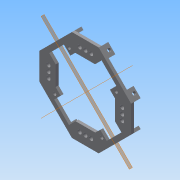
# Autodesk Inventor part: fix_board
Saved by Autodesk Inventor 2015 (Build 190159000, 159)
## iProperties
Created: 2015-06-18
Part Number: fix_board
Material: Générique
Document SubType Name: Modeling
Designer: Gregwar
Density: 1 g/cm^3
Appearance: Par défaut
Author: Gregwar
Autodesk Inventor part; units mm, degrees
note: some values were not read from the file. Chosen so that the rebuilt part matches the saved one: second side of "Extrusion3".
ref_plane "YZ Plane" through (0, 0, 0) normal (1, 0, 0) x (0, 1, 0)
ref_plane "XZ Plane" through (0, 0, 0) normal (0, 1, 0) x (-1, 0, 0)
ref_plane "XY Plane" through (0, 0, 0) normal (0, 0, 1) x (1, 0, 0)
sketch "Esquisse1" plane through (0, 0, 0) normal (0, 1, 0) x (-1, 0, 0)
  line L0 (35, 35) -> (35, 14)
  line L1 (35, 14) -> (42, 10)
  line L2 (42, 10) -> (42, 0)
  line L3 (35, 35) -> (0, 0)
  line L4 (42, 0) -> (0, 0) construction
  line L5 (35, -35) -> (35, -14)
  line L6 (35, -14) -> (42, -10)
  line L7 (42, -10) -> (42, 0)
  line L8 (35, -35) -> (0, 0)
  line L9 (38.5, -12) -> (38.5, 12) construction
  circle A0 centre (38.5, 0) radius 2.15
  circle A1 centre (38.5, 6) radius 2.15
  circle A2 centre (38.5, -6) radius 2.15
  dimension "d0" = 90
  dimension "d1" = 70
  dimension "d4" = 6
  dimension "d11" = 6
  dimension "d16" = 4.3
  dimension "d17" = 20
  dimension "d18" = 4
  dimension "d19" = 7
  constraints: 20 end point, 3 centre point, 3 midpoint, 3 symmetric about line, 3 vertical, 1 horizontal, 1 parallel, 4 other
  measures "d0" angle of L3 L8
  measures "d1" distance of L0.start L5.start
  measures "d4" distance of A0.centre A1.centre
  measures "d11" distance of A0.centre A2.centre
  measures "d16" diameter of A0
  measures "d17" distance of L1.end L6.end
  measures "d18" vertical distance of L1.end L0.end
  measures "d19" distance between parallel lines of L5 L7
extrude "Extrusion1" add sketch "Esquisse1" along normal blind 3
pattern_circular "Réseau circulaire1" count 4 over 360 about axis through (0, 0, 0) along (0, 1, 0) of "Extrusion1"
chamfer "Chanfrein1" distance 8 angle 45 4 edges at (35, 1.5, -35) (-35, 1.5, -35) (-35, 1.5, 35) (35, 1.5, 35)
ref_plane "Plan de construction3" through (-4, 0, 4) normal (0.7071068, 0, 0.7071068) x (0.7071068, 0, -0.7071068)
ref_plane "Plan de construction4" through (-4, 0, -4) normal (-0.7071068, 0, 0.7071068) x (0.7071068, 0, 0.7071068)
sketch "Esquisse3" plane through (0, 0, 0) normal (0, -1, 0) x (1, 0, 0)
  circle A0 centre (0, 38.5) radius 2.15 projected
  circle A1 centre (6, 38.5) radius 2.15 projected
  circle A2 centre (-6, 38.5) radius 2.15 projected
  circle A3 centre (38.5, 6) radius 2.15 projected
  circle A4 centre (38.5, -6) radius 2.15 projected
  circle A5 centre (38.5, 0) radius 2.15 projected
  circle A6 centre (6, -38.5) radius 2.15 projected
  circle A7 centre (-6, -38.5) radius 2.15 projected
  circle A8 centre (0, -38.5) radius 2.15 projected
  circle A9 centre (-38.5, -6) radius 2.15 projected
  circle A10 centre (-38.5, 6) radius 2.15 projected
  circle A11 centre (-38.5, 0) radius 2.15 projected
  line L0 (27, 35) -> (35, 27) projected
  line L1 (27, 35) -> (14, 35) projected
  line L2 (14, 35) -> (10, 42) projected
  line L3 (10, 42) -> (-10, 42) projected
  line L4 (-10, 42) -> (-14, 35) projected
  line L5 (-14, 35) -> (-27, 35) projected
  line L6 (-35, 27) -> (-27, 35) projected
  line L7 (-35, 27) -> (-35, 14) projected
  line L8 (-35, 14) -> (-42, 10) projected
  line L9 (-42, 10) -> (-42, -10) projected
  line L10 (-42, -10) -> (-35, -14) projected
  line L11 (-35, -14) -> (-35, -27) projected
  line L12 (-27, -35) -> (-35, -27) projected
  line L13 (-27, -35) -> (-14, -35) projected
  line L14 (-14, -35) -> (-10, -42) projected
  line L15 (-10, -42) -> (10, -42) projected
  line L16 (10, -42) -> (14, -35) projected
  line L17 (14, -35) -> (27, -35) projected
  line L18 (35, -27) -> (27, -35) projected
  line L19 (35, -27) -> (35, -14) projected
  line L20 (35, -14) -> (42, -10) projected
  line L21 (42, -10) -> (42, 10) projected
  line L22 (42, 10) -> (35, 14) projected
  line L23 (35, 14) -> (35, 27) projected
  line L24 (-47.9706, 14.0294) -> (-14.0294, 47.9706)
  line L25 (-14.0294, 47.9706) -> (-11.9081, 45.8492)
  line L26 (-11.9081, 45.8492) -> (-45.8492, 11.9081)
  line L27 (-45.8492, 11.9081) -> (-47.9706, 14.0294)
  point P0 (0, 0)
  point P1 (-31, 31)
  dimension "d35" = 48
  dimension "d36" = 3
  constraints: 8 end point, 2 midpoint, 2 perpendicular, 1 collinear, 1 parallel
  measures "d35" distance of L24.start L24.end
  measures "d36" distance of L24.end L25.end
extrude "Extrusion3" add sketch "Esquisse3" against normal blind 10 contours L26 L7 L6 L5 | L5 L24 L25 L26 | L26 L27 L24 L7
sketch "Esquisse4" plane through (-14.0294, 0, 47.9706) normal (-0.7071068, 0, 0.7071068) x (0.7071068, 0, 0.7071068)
  line L0 (0, 0) -> (-48, 0) projected
  line L1 (0, 0) -> (0, 10) projected
  line L2 (-48, 10) -> (0, 10) projected
  line L3 (-48, 0) -> (-48, 10) projected
  line L4 (-48, 0) -> (-48, 10) construction
  line L5 (-48, 7) -> (0, 7) construction
  line L6 (0, 0) -> (0, 10) construction
  circle A0 centre (-42.5, 7) radius 1.75
  line L7 (0, 10) -> (-48, 10) construction
  line L8 (-24, 10) -> (-24, 0) construction
  circle A1 centre (-5.5, 7) radius 1.75
  dimension "d41" = 10
  dimension "d42" = 3
  dimension "d43" = 37
  dimension "d44" = 3.5
  constraints: 4 end point, 3 point on line, 2 centre point, 1 horizontal, 1 midpoint, 1 symmetric about line, 1 vertical, 1 other
  measures "d41" distance between parallel lines of L0 L2
  measures "d42" distance between parallel lines of L5 L2
  measures "d43" distance of A0.centre A1.centre
  measures "d44" diameter of A0
extrude "Extrusion4" cut sketch "Esquisse4" against normal through all contours A0 | A1
sketch "Esquisse6" plane through (-14.0294, 0, 47.9706) normal (-0.7071068, 0, 0.7071068) x (0.7071068, 0, 0.7071068)
  line L0 (-15.3431, 3) -> (-9.1508, 3) projected
  circle A0 centre (-5.5, 7) radius 1.75 projected
  circle A1 centre (-42.5, 7) radius 1.75 projected
  line L1 (0, 0) -> (-48, 0) projected
  line L2 (0, 0) -> (0, 10) projected
  line L3 (-48, 10) -> (0, 10) projected
  line L4 (-48, 0) -> (-48, 10) projected
  line L5 (-10.5, 10) -> (-37.5, 10)
  line L6 (-37.5, 10) -> (-37.5, 3)
  line L7 (-37.5, 3) -> (-10.5, 3)
  line L8 (-10.5, 3) -> (-10.5, 10)
  point P0 (-24, 0)
  point P1 (-24, 10)
  dimension "d51" = 27
  dimension "d63" = 3
  constraints: 8 end point, 2 midpoint, 2 parallel, 1 horizontal, 1 perpendicular
  measures "d51" distance of L6.end L7.end
  measures "d63" distance between parallel lines of L7 L1
extrude "Extrusion5" cut sketch "Esquisse6" against normal through all contours L7 L6 L3 L8 L0
pattern_circular "Réseau circulaire5" count 4 over 360 about axis through (0, 0, 0) along (0, 1, 0) of "Extrusion3", "Extrusion4", "Extrusion5"
sketch "Esquisse11" plane through (0, 0, 0) normal (0, -1, 0) x (1, 0, 0)
  circle A0 centre (0, 38.5) radius 2.15 construction
  circle A1 centre (6, 38.5) radius 2.15 construction
  circle A2 centre (-6, 38.5) radius 2.15 construction
  circle A3 centre (38.5, 6) radius 2.15 construction
  circle A4 centre (38.5, -6) radius 2.15 construction
  circle A5 centre (38.5, 0) radius 2.15 construction
  circle A6 centre (6, -38.5) radius 2.15 construction
  circle A7 centre (-6, -38.5) radius 2.15 construction
  circle A8 centre (0, -38.5) radius 2.15 construction
  circle A9 centre (-38.5, -6) radius 2.15 construction
  circle A10 centre (-38.5, 6) radius 2.15 construction
  circle A11 centre (-38.5, 0) radius 2.15 construction
  line L0 (-22.7574, -35) -> (-14, -35) construction
  line L1 (-14, -35) -> (-10, -42) construction
  line L2 (-10, -42) -> (10, -42) construction
  line L3 (10, -42) -> (14, -35) construction
  line L4 (14, -35) -> (22.7574, -35) construction
  line L5 (22.7574, -35) -> (11.9081, -45.8492) construction
  line L6 (11.9081, -45.8492) -> (14.0294, -47.9706) construction
  line L7 (14.0294, -47.9706) -> (47.9706, -14.0294) construction
  line L8 (47.9706, -14.0294) -> (45.8492, -11.9081) projected
  line L9 (45.8492, -11.9081) -> (35, -22.7574) projected
  line L10 (35, -22.7574) -> (35, -14) projected
  line L11 (35, -14) -> (42, -10) projected
  line L12 (42, -10) -> (42, 10) projected
  line L13 (42, 10) -> (35, 14) projected
  line L14 (35, 14) -> (35, 22.7574) projected
  line L15 (35, 22.7574) -> (45.8492, 11.9081) projected
  line L16 (45.8492, 11.9081) -> (47.9706, 14.0294) projected
  line L17 (47.9706, 14.0294) -> (14.0294, 47.9706) construction
  line L18 (14.0294, 47.9706) -> (11.9081, 45.8492) construction
  line L19 (11.9081, 45.8492) -> (22.7574, 35) construction
  line L20 (22.7574, 35) -> (14, 35) construction
  line L21 (14, 35) -> (10, 42) construction
  line L22 (10, 42) -> (-10, 42) construction
  line L23 (-10, 42) -> (-14, 35) construction
  line L24 (-14, 35) -> (-22.7574, 35) construction
  line L25 (-22.7574, 35) -> (-11.9081, 45.8492) construction
  line L26 (-11.9081, 45.8492) -> (-14.0294, 47.9706) construction
  line L27 (-14.0294, 47.9706) -> (-47.9706, 14.0294) construction
  line L28 (-47.9706, 14.0294) -> (-45.8492, 11.9081) construction
  line L29 (-45.8492, 11.9081) -> (-35, 22.7574) construction
  line L30 (-35, 22.7574) -> (-35, 14) construction
  line L31 (-35, 14) -> (-42, 10) construction
  line L32 (-42, 10) -> (-42, -10) construction
  line L33 (-42, -10) -> (-35, -14) construction
  line L34 (-35, -14) -> (-35, -22.7574) construction
  line L35 (-35, -22.7574) -> (-45.8492, -11.9081) construction
  line L36 (-45.8492, -11.9081) -> (-47.9706, -14.0294) construction
  line L37 (-47.9706, -14.0294) -> (-14.0294, -47.9706) construction
  line L38 (-14.0294, -47.9706) -> (-11.9081, -45.8492) construction
  line L39 (-11.9081, -45.8492) -> (-22.7574, -35) construction
  line L40 (47.9706, -14.0294) -> (47.9706, 14.0294)
  point P0 (0, 0)
  constraints: 2 end point, 1 vertical
extrude "Extrusion8" add sketch "Esquisse11" against normal blind 3
pattern_circular "Réseau circulaire6" count 4 over 360 about axis through (0, 0, 0) along (0, 1, 0) of "Extrusion8"
sketch "Esquisse9" plane through (0, 0, 0) normal (0, -1, 0) x (1, 0, 0)
  line L0 (0, 0) -> (21.8388, 21.8388) construction
  line L1 (0, 0) -> (66.7346, 0) construction
  line L2 (0, 0) -> (0, 22.6965) construction
  line L3 (31.4289, 0) -> (31.4289, 10)
  line L4 (31.4289, 10) -> (38.5, 17.0711)
  line L5 (38.5, 17.0711) -> (27.7855, 27.7855)
  line L6 (0, 31.4289) -> (10, 31.4289)
  line L7 (10, 31.4289) -> (17.0711, 38.5)
  line L8 (17.0711, 38.5) -> (27.7855, 27.7855)
  line L9 (38.5, -17.0711) -> (27.7855, -27.7855)
  line L10 (31.4289, -10) -> (38.5, -17.0711)
  line L11 (31.4289, 0) -> (31.4289, -10)
  line L12 (17.0711, -38.5) -> (27.7855, -27.7855)
  line L13 (10, -31.4289) -> (17.0711, -38.5)
  line L14 (0, -31.4289) -> (10, -31.4289)
  line L15 (-31.4289, 0) -> (-31.4289, -10)
  line L16 (-31.4289, -10) -> (-38.5, -17.0711)
  line L17 (-38.5, -17.0711) -> (-27.7855, -27.7855)
  line L18 (-17.0711, -38.5) -> (-27.7855, -27.7855)
  line L19 (0, -31.4289) -> (-10, -31.4289)
  line L20 (-10, -31.4289) -> (-17.0711, -38.5)
  line L21 (0, 0) -> (-66.7346, 0) construction
  line L22 (-31.4289, 0) -> (-31.4289, 10)
  line L23 (-31.4289, 10) -> (-38.5, 17.0711)
  line L24 (0, 31.4289) -> (-10, 31.4289)
  line L25 (0, 0) -> (-21.8388, 21.8388) construction
  line L26 (-10, 31.4289) -> (-17.0711, 38.5)
  line L27 (-17.0711, 38.5) -> (-27.7855, 27.7855)
  line L28 (-38.5, 17.0711) -> (-27.7855, 27.7855)
  line L29 (27.432, 27.432) -> (37.7929, 17.0711)
  line L30 (37.7929, 17.0711) -> (30.9289, 10.2071)
  line L31 (30.9289, 10.2071) -> (30.9289, 0)
  line L32 (30.9289, 0) -> (30.9289, -10.2071)
  line L33 (30.9289, -10.2071) -> (37.7929, -17.0711)
  line L34 (37.7929, -17.0711) -> (27.432, -27.432)
  line L35 (27.432, -27.432) -> (17.0711, -37.7929)
  line L36 (17.0711, -37.7929) -> (10.2071, -30.9289)
  line L37 (10.2071, -30.9289) -> (0, -30.9289)
  line L38 (0, -30.9289) -> (-10.2071, -30.9289)
  line L39 (-10.2071, -30.9289) -> (-17.0711, -37.7929)
  line L40 (-17.0711, -37.7929) -> (-27.432, -27.432)
  line L41 (-27.432, -27.432) -> (-37.7929, -17.0711)
  line L42 (-37.7929, -17.0711) -> (-30.9289, -10.2071)
  line L43 (-30.9289, -10.2071) -> (-30.9289, 0)
  line L44 (-30.9289, 0) -> (-30.9289, 10.2071)
  line L45 (-30.9289, 10.2071) -> (-37.7929, 17.0711)
  line L46 (-37.7929, 17.0711) -> (-27.432, 27.432)
  line L47 (-27.432, 27.432) -> (-17.0711, 37.7929)
  line L48 (-17.0711, 37.7929) -> (-10.2071, 30.9289)
  line L49 (-10.2071, 30.9289) -> (0, 30.9289)
  line L50 (0, 30.9289) -> (10.2071, 30.9289)
  line L51 (10.2071, 30.9289) -> (17.0711, 37.7929)
  line L52 (17.0711, 37.7929) -> (27.432, 27.432)
  dimension "d67" = 45
  dimension "d68" = 10
  dimension "d69" = 10
  dimension "d70" = 38.5
  dimension "d71" = 77
  dimension "d86" = 0.5
  constraints: 106 end point, 22 symmetric about line, 4 point on line, 2 collinear, 2 parallel, 2 vertical, 1 coincident, 1 horizontal, 23 other
  measures "d67" angle of L0 L1
  measures "d68" distance of L3.start L3.end
  measures "d69" distance of L3.end L5.start
  measures "d70" distance from line of L1 L7.end
  measures "d71" distance of L13.end L7.end
  measures "d86" distance between parallel lines of L5 L29
extrude "Extrusion9" cut sketch "Esquisse9" against normal through all contours L29 L30 L31 L32 L33 L34 L35 L36 L37 L38 L39 L40 L41 L42 L43 L44 L45 L46 L47 L48 L49 L50 L51 L52
sketch "Esquisse12" plane through (0, 3, 0) normal (0, 1, 0) x (1, 0, 0)
  line L0 (-10, -31.4289) -> (-17.0711, -38.5) projected
  line L1 (-17.0711, -38.5) -> (-27.7855, -27.7855) projected
  line L2 (-31.4289, -10) -> (-38.5, -17.0711) projected
  line L3 (-38.5, -17.0711) -> (-27.7855, -27.7855) projected
  line L4 (-10, -31.4289) -> (-15.6569, -25.7721)
  line L5 (-15.6569, -25.7721) -> (-22.7279, -32.8431)
  circle A0 centre (-17.0711, -32.136) radius 1.75
  line L6 (-10, -31.4289) -> (-17.0711, -38.5)
  line L7 (-17.0711, -38.5) -> (-22.7279, -32.8431)
  line L8 (31.4289, -10) -> (25.7721, -15.6569)
  line L9 (25.7721, -15.6569) -> (32.8431, -22.7279)
  circle A1 centre (32.136, -17.0711) radius 1.75
  line L10 (31.4289, -10) -> (38.5, -17.0711)
  line L11 (38.5, -17.0711) -> (32.8431, -22.7279)
  line L12 (10, 31.4289) -> (15.6569, 25.7721)
  line L13 (15.6569, 25.7721) -> (22.7279, 32.8431)
  circle A2 centre (17.0711, 32.136) radius 1.75
  line L14 (10, 31.4289) -> (17.0711, 38.5)
  line L15 (17.0711, 38.5) -> (22.7279, 32.8431)
  line L16 (-31.4289, 10) -> (-25.7721, 15.6569)
  line L17 (-25.7721, 15.6569) -> (-32.8431, 22.7279)
  circle A3 centre (-32.136, 17.0711) radius 1.75
  line L18 (-31.4289, 10) -> (-38.5, 17.0711)
  line L19 (-38.5, 17.0711) -> (-32.8431, 22.7279)
  point P0 (0, 0)
  dimension "d89" = 4.5
  dimension "d90" = 4.5
  dimension "d91" = 3.5
  dimension "d94" = 360
  dimension "d98" = 8
  constraints: 32 end point, 4 centre point, 2 perpendicular, 1 collinear, 1 point on line, 41 other
  measures "d89" distance from line of L0 A0.centre
  measures "d90" distance from line of L1 A0.centre
  measures "d91" diameter of A0
  measures "d98" distance between parallel lines of L0 L5
extrude "Extrusion10" add sketch "Esquisse12" against normal blind 3
